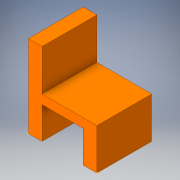
# Autodesk Inventor part: Sun_Base
Saved by Autodesk Inventor 2016 (Build 200138000, 138)
## iProperties
Created: 2017-10-05
Part Number: Sun_Base
Material: Generic
Document SubType Name: Sheet Metal
Designer: sun01147
Density: 1 g/cm^3
Sheet Metal Rule: Default
Appearance: Default
Author: sun01147
Autodesk Inventor part; units mm, degrees
ref_plane "YZ Plane" through (0, 0, 0) normal (1, 0, 0) x (0, 1, 0)
ref_plane "XZ Plane" through (0, 0, 0) normal (0, 1, 0) x (-1, 0, 0)
ref_plane "XY Plane" through (0, 0, 0) normal (0, 0, 1) x (1, 0, 0)
sketch "Sketch1" plane through (0, 0, 0) normal (0, 0, 1) x (1, 0, 0)
  line L0 (0, 38.1) -> (0, 0)
  line L1 (0, 0) -> (6.35, 0)
  line L2 (0, 38.1) -> (6.35, 38.1)
  line L3 (6.35, 38.1) -> (6.35, 19.05)
  line L4 (6.35, 19.05) -> (31.75, 19.05)
  line L5 (6.35, 0) -> (6.35, 14.7925)
  line L6 (31.75, 19.05) -> (31.75, 0)
  line L7 (31.75, 0) -> (25.4, 0)
  line L8 (6.35, 14.7925) -> (6.35, 19.05)
  line L9 (25.4, 0) -> (25.4, 14.7925)
  line L10 (25.4, 14.7925) -> (6.35, 14.7925)
  line L11 (25.4, 14.7925) -> (31.75, 14.7925)
  dimension "d0" = 38.1
  dimension "d1" = 6.35
  dimension "d2" = 6.35
  dimension "d3" = 19.05
  dimension "d4" = 25.4
  dimension "d7" = 6.35
  constraints: 24 end point, 5 vertical, 3 horizontal, 2 perpendicular, 2 point on line
  measures "d0" distance of L0.start L0.end
  measures "d1" distance of L0.start L2.end
  measures "d2" distance of L0.end L1.end
  measures "d3" distance of L2.end L3.end
  measures "d4" distance of L3.end L4.end
  measures "d7" distance of L6.end L7.end
sketch "Sketch2" plane through (0, 0, 0) normal (0, 0, 1) x (1, 0, 0)
  point P0 (0, 0)
extrude "Extrusion1" add sketch "Sketch1" against normal blind 25.4
sketch "Sketch3" plane through (0, 0, 0) normal (0, 0, 1) x (1, 0, 0)
  point P0 (0, 0)
sketch "Sketch4" plane through (31.75, 0, 0) normal (1, 0, 0) x (0, 0, -1)
  point P0 (0, 0)
equation "\"BendRadius\" = Thickness"
equation "\"BendReliefWidth\" = Thickness"
equation "\"BendReliefDepth\" = 0.5 * Thickness"
equation "\"CornerReliefSize\" = 4 * Thickness"
equation "\"MinimumRemnant\" = 2 * Thickness"
equation "\"TransitionRadius\" = BendRadius"
equation "\"JacobiRadiusSize\" = BendRadius"
equation "\"GapSize\" = Thickness"
equation "\"Thickness\" = 3.048"
body "Solid1"
